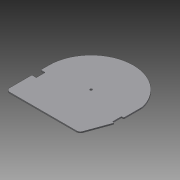
# Autodesk Inventor part: PT Flange Outer
Saved by Autodesk Inventor 2015 (Build 190159000, 159)
## iProperties
Created: 2015-06-18
Part Number: PT Flange Outer
Material: Generic
Document SubType Name: Modeling
Designer: JR
Density: 1 g/cm^3
Appearance: Default
Author: JR
Autodesk Inventor part; units mm, degrees
ref_plane "YZ Plane" through (0, 0, 0) normal (1, 0, 0) x (0, 1, 0)
ref_plane "XZ Plane" through (0, 0, 0) normal (0, 1, 0) x (-1, 0, 0)
ref_plane "XY Plane" through (0, 0, 0) normal (0, 0, 1) x (1, 0, 0)
sketch "Sketch1" plane through (0, 0, 0) normal (0, 0, 1) x (1, 0, 0)
  circle A0 centre (0, 0) radius 1.5
  arc A1 (53.9189, 18.4865) -> (-57, 0) centre (0, 0) ccw
  arc A2 (55, 12) -> (53.9189, 18.4865) centre (35, 12) ccw
  line L0 (55, 12) -> (55, -11)
  line L1 (55, -11) -> (52, -11)
  line L2 (52, -11) -> (52, -23)
  line L3 (52, -23) -> (54.739, -23)
  line L4 (54.739, -23) -> (42, -58)
  line L5 (42, -58) -> (-57, -58)
  line L6 (-57, -58) -> (-57, -23)
  line L7 (-57, -23) -> (-51, -23)
  line L8 (-51, -23) -> (-51, -11)
  line L9 (-51, -11) -> (-57, -11)
  line L10 (-57, 0) -> (-57, -11)
  dimension "d0" = 3
  dimension "d1" = 57
  dimension "d2" = 20
  dimension "d3" = 6
  dimension "d4" = 12
  dimension "d5" = 55
  dimension "d6" = 3
  dimension "d7" = 110
  dimension "d8" = 99
  dimension "d9" = 47
  dimension "d10" = 58
  constraints: 22 end point, 6 perpendicular, 5 point on line, 4 point on circle, 3 centre point, 3 tangent, 1 coincident, 1 concentric, 1 parallel, 1 vertical
  measures "d0" diameter of A0
  measures "d1" radius of A1
  measures "d2" radius of A2
  measures "d3" distance of L6.end L7.end
  measures "d4" distance of L1.end L2.end
  measures "d5" distance from line of L0 point (0, 0)
  measures "d6" distance of L0.end L1.end
  measures "d7" angle of L5 L4
  measures "d8" distance of L4.end L5.end
  measures "d9" distance between parallel lines of L5 L9
  measures "d10" distance from line of L5 point (0, 0)
extrude "Extrusion1" add sketch "Sketch1" along normal blind 1.5
fillet "Fillet1" radius 0.5 4 edges at (52, -11, 0.75) (52, -23, 0.75) (-51, -11, 0.75) (-51, -23, 0.75)
fillet "Fillet2" radius 1 4 edges at (-57, -11, 0.75) (-57, -23, 0.75) (54.739, -23, 0.75) (55, -11, 0.75)
fillet "Fillet3" radius 5 2 edges at (42, -58, 0.75) (-57, -58, 0.75)
body "Solid1"
